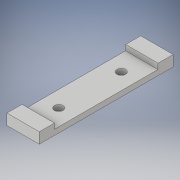
# Autodesk Inventor part: joint1_gear_holder
Saved by Autodesk Inventor 2019 (Build 230136000, 136)
## iProperties
Created: 2019-12-26
Part Number: joint1_gear_holder
Material: Типовые
Document SubType Name: Modeling
Designer: Петров Иван
Density: 1 g/cm^3
Appearance: По умолчанию
Author: Петров Иван
Autodesk Inventor part; units mm, degrees
ref_plane "YZ Plane" through (0, 0, 0) normal (1, 0, 0) x (0, 1, 0)
ref_plane "XZ Plane" through (0, 0, 0) normal (0, 1, 0) x (-1, 0, 0)
ref_plane "XY Plane" through (0, 0, 0) normal (0, 0, 1) x (1, 0, 0)
sketch "Эскиз1" plane through (0, 0, 0) normal (0, 1, 0) x (-1, 0, 0)
  line L0 (-15, 62) -> (15, 62)
  line L1 (15, 62) -> (15, -62)
  line L2 (15, -62) -> (-15, -62)
  line L3 (-15, -62) -> (-15, 62)
  line L4 (-15, 62) -> (15, -62) construction
  line L5 (15, 62) -> (-15, -62) construction
  point P0 (0, 0)
  dimension "d0" = 30
  dimension "d1" = 124
  constraints: 12 end point, 2 midpoint, 2 parallel, 1 horizontal, 1 perpendicular
  measures "d0" distance of L1.end L2.end
  measures "d1" distance of L0.end L1.end
extrude "Выдавливание1" add sketch "Эскиз1" along normal blind 5
sketch "Эскиз2" plane through (0, 5, 0) normal (0, 1, 0) x (1, 0, 0)
  line L0 (-15, -62) -> (15, -62) projected
  line L1 (15, -62) -> (15, 62) projected
  line L2 (-15, -62) -> (15, -62)
  line L3 (15, -62) -> (15, -48)
  line L4 (15, -48) -> (-15, -48)
  line L5 (-15, -48) -> (-15, -62)
  point P0 (0, 0)
  dimension "d4" = 14
  constraints: 8 end point, 2 parallel, 1 horizontal, 1 perpendicular, 1 point on line
  measures "d4" distance of L3.end L2.end
extrude "Выдавливание2" add sketch "Эскиз2" along normal blind 5
mirror "Зеркальное отражение1" about plane through (0, 0, 0) normal (0, 0, 1) of "Выдавливание2"
sketch "Эскиз3" plane through (0, 5, 0) normal (0, 1, 0) x (1, 0, 0)
  line L0 (15, 48) -> (-15, 48) projected
  line L1 (0, 48) -> (0, 29)
  circle A0 centre (0, 29) radius 4
  point P0 (0, 0)
  dimension "d7" = 19
  dimension "d8" = 8
  constraints: 2 end point, 1 centre point, 1 coincident, 1 midpoint, 1 vertical
  measures "d7" distance of L1.start L1.end
  measures "d8" diameter of A0
extrude "Выдавливание3" cut sketch "Эскиз3" against normal blind 15
mirror "Зеркальное отражение2" about plane through (0, 0, 0) normal (0, 0, 1) of "Выдавливание3"
